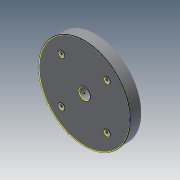
# Autodesk Inventor part: drivepullySide
Saved by Autodesk Inventor 2015 (Build 190159000, 159)
## iProperties
Created: 2014-09-01
Part Number: drivepullySide
Material: Generic
Document SubType Name: Modeling
Designer: shohei
Density: 1 g/cm^3
Appearance: Default
Author: shohei
Autodesk Inventor part; units mm, degrees
ref_plane "YZ Plane" through (0, 0, 0) normal (1, 0, 0) x (0, 1, 0)
ref_plane "XZ Plane" through (0, 0, 0) normal (0, 1, 0) x (-1, 0, 0)
ref_plane "XY Plane" through (0, 0, 0) normal (0, 0, 1) x (1, 0, 0)
sketch "Block1" plane through (0, 0, 0) normal (0, 0, 1) x (1, 0, 0)
  circle A0 centre (0, 0) radius 60.22
  circle A1 centre (-30, -30) radius 2.72
  circle A2 centre (30, -30) radius 2.72
  circle A3 centre (0, 0) radius 5.22
  circle A4 centre (-30, 30) radius 2.72
  circle A5 centre (30, 30) radius 2.72
sketch "Block2" plane through (0, 0, 0) normal (0, 0, 1) x (1, 0, 0)
  circle A0 centre (0, 0) radius 40.22
  circle A1 centre (20, 20) radius 2.72
  circle A2 centre (-20, 20) radius 2.72
  circle A3 centre (0, 0) radius 5.22
  circle A4 centre (20, -20) radius 2.72
  circle A5 centre (-20, -20) radius 2.72
sketch "Sketch1" plane through (0, 0, 0) normal (0, 1, 0) x (-1, 0, 0)
  circle A0 centre (0, 0) radius 40
  circle A1 centre (0, 0) radius 5
  circle A2 centre (20, 20) radius 2.5
  line L0 (84.308, 0) -> (-84.308, 0) projected
  line L1 (0, -84.308) -> (0, 84.308) projected
  circle A3 centre (20, -20) radius 2.5
  circle A4 centre (-20, 20) radius 2.5
  circle A5 centre (-20, -20) radius 2.5
  dimension "d0" = 80
  dimension "d3" = 10
  dimension "d6" = 5
  dimension "d7" = 20
  dimension "d8" = 20
  constraints: 6 centre point, 3 symmetric about line, 2 coincident, 3 other
  measures "d0" diameter of A0
  measures "d3" diameter of A1
  measures "d6" diameter of A2
  measures "d7" distance from line of L1 A2.centre
  measures "d8" distance from line of L0 A2.centre
extrude "Extrusion3" add sketch "Sketch1" along normal blind 10 contours L0 A1 L1 A0 | A0 L1 A1 L0 | L1 A1 L0 A0 | A0 L0 A1 L1
sketch "Sketch4" plane through (0, 0, 0) normal (0, -1, 0) x (1, 0, 0)
  circle A0 centre (0, 0) radius 5 projected
  circle A1 centre (20, 20) radius 2.5 projected
  circle A2 centre (20, -20) radius 2.5 projected
  circle A3 centre (-20, -20) radius 2.5 projected
  circle A4 centre (-20, 20) radius 2.5 projected
  circle A5 centre (0, 0) radius 40 projected
  circle A6 centre (0, 0) radius 40.22
  circle A7 centre (20, 20) radius 2.72
  circle A8 centre (-20, 20) radius 2.72
  circle A9 centre (0, 0) radius 5.22
  circle A10 centre (20, -20) radius 2.72
  circle A11 centre (-20, -20) radius 2.72
  constraints: 6 other
sketch "Sketch5" plane through (0, 0, 0) normal (0, 1, 0) x (-1, 0, 0)
  circle A0 centre (0, 0) radius 40.22
  circle A1 centre (20, 20) radius 2.72
  circle A2 centre (-20, 20) radius 2.72
  circle A3 centre (0, 0) radius 5.22
  circle A4 centre (20, -20) radius 2.72
  circle A5 centre (-20, -20) radius 2.72
body "Solid3"
